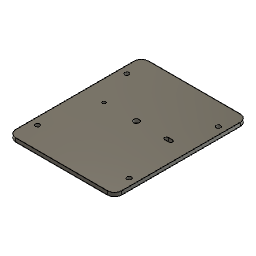
halteplatte_lidart v2 (Autodesk Fusion 360 design; units mm, degrees)
Autodesk Fusion 360 part; units mm, degrees
note: some values were not read from the file. Set by a fixed rule: which sketch regions a step uses.
sketch "Skizze1" plane through (0, 0, 0) normal (0, 1, 0) x (1, 0, 0)
  line L0 (10, 0) -> (136, 0)
  line L1 (146, -10) -> (146, -173)
  line L2 (136, -183) -> (10, -183)
  line L3 (0, -173) -> (0, -10)
  line L4 (20, -20) -> (126, -20)
  line L5 (126, -20) -> (126, -163)
  line L6 (126, -163) -> (20, -163)
  line L7 (20, -163) -> (20, -20)
  circle A0 centre (10, -30) radius 3
  circle A1 centre (10, -153) radius 3
  circle A2 centre (136, -30) radius 3
  circle A3 centre (136, -153) radius 3
  circle A4 centre (28.55, -80) radius 2.25
  line L8 (120.45, -77.5) -> (114.45, -77.5)
  arc A5 (114.45, -77.5) -> (114.45, -82.5) centre (114.45, -80) ccw
  line L9 (114.45, -82.5) -> (120.45, -82.5)
  arc A6 (120.45, -82.5) -> (120.45, -77.5) centre (120.45, -80) ccw
  line L10 (120.45, -80) -> (114.45, -80) construction
  circle A7 centre (73, -80) radius 4
  arc A8 (10, 0) -> (0, -10) centre (10, -10) ccw
  arc A9 (146, -10) -> (136, 0) centre (136, -10) ccw
  arc A10 (0, -173) -> (10, -183) centre (10, -173) ccw
  arc A11 (136, -183) -> (146, -173) centre (136, -173) ccw
  point P0 (146, 0)
  point P1 (0, -183)
  point P2 (117.45, -80)
  dimension "d1" = 183
  dimension "d2" = 146
  dimension "d3" = 20
  dimension "d4" = 20
  dimension "d5" = 20
  dimension "d6" = 20
  dimension "d7" = 6
  dimension "d8" = 6
  dimension "d9" = 6
  dimension "d10" = 6
  dimension "d11" = 10
  dimension "d12" = 10
  dimension "d13" = 30
  dimension "d14" = 30
  dimension "d15" = 30
  dimension "d16" = 10
  dimension "d17" = 10
  dimension "d18" = 30
  dimension "d19" = 4.5
  dimension "d22" = 8.55
  dimension "d24" = 6
  dimension "d25" = 5
  dimension "d26" = 88.9
  dimension "d27" = 60
  dimension "d28" = 60
  dimension "d30" = 8
  dimension "d31" = 44.45
  dimension "d32" = 60
  dimension "d35" = 10
  constraint horizontal L0
  constraint vertical L1
  constraint horizontal L2
  constraint vertical L3
  constraint horizontal L4
  constraint vertical L5
  constraint horizontal L6
  constraint vertical L7
  constraint tangent L8 A5
  constraint tangent A5 L9
  constraint parallel L8 L9
  constraint tangent L9 A6
  constraint tangent L8 A6
  constraint horizontal L10
  constraint midpoint L10 P2
  constraint coincident origin L0
  constraint coincident origin L3
  constraint tangent L0 A8
  constraint tangent L3 A8
  constraint coincident P0 L0
  constraint coincident P0 L1
  constraint tangent L0 A9
  constraint tangent L1 A9
  constraint equal A8 A9
  constraint coincident P1 L2
  constraint coincident P1 L3
  constraint tangent L2 A10
  constraint tangent L3 A10
  constraint equal A8 A10
  constraint tangent L1 A11
  constraint tangent L2 A11
  constraint equal A8 A11
  measures "d1" distance of origin P1
  measures "d2" distance of origin P0
  measures "d3" distance of L3 L7
  measures "d4" distance of L1 L5
  measures "d5" distance of L0 L4
  measures "d6" distance of L2 L6
  measures "d7" diameter of A0
  measures "d8" diameter of A1
  measures "d9" diameter of A2
  measures "d10" diameter of A3
  measures "d11" distance of L3 A0.centre
  measures "d12" distance of L3 A1.centre
  measures "d13" distance of L2 A1.centre
  measures "d14" distance of L0 A0.centre
  measures "d15" distance of L0 A2.centre
  measures "d16" distance of L1 A2.centre
  measures "d17" distance of L1 A3.centre
  measures "d18" distance of L2 A3.centre
  measures "d19" diameter of A4
  measures "d22" distance of L7 A4.centre
  measures "d24" distance of A6.centre A5.centre
  measures "d25" distance of L8 L9
  measures "d26" horizontal distance of A4.centre P2
  measures "d27" distance of L4 A4.centre
  measures "d28" distance of L4 P2
  measures "d30" diameter of A7
  measures "d31" horizontal distance of A4.centre A7.centre
  measures "d32" distance of L4 A7.centre
  measures "d35" radius of A8 A9
extrude "Extrusion1" add sketch "Skizze1" along normal blind 5 contours L0 L1 L2 L3 A8 A9 A10 A11 | L4 L5 L6 L7
